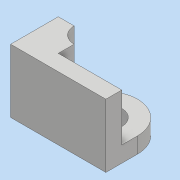
# Autodesk Inventor part: 7
Saved by Autodesk Inventor 2017 (Build 210142000, 142)
## iProperties
Part Number: 7
Material: 一般
Document SubType Name: Modeling
Designer: d8910
Density: 1 g/cm^3
Appearance: 預設
Author: d8910
Autodesk Inventor part; units mm, degrees
ref_plane "YZ Plane" through (0, 0, 0) normal (1, 0, 0) x (0, 1, 0)
ref_plane "XZ Plane" through (0, 0, 0) normal (0, 1, 0) x (-1, 0, 0)
ref_plane "XY Plane" through (0, 0, 0) normal (0, 0, 1) x (1, 0, 0)
sketch "草圖1" plane through (0, 0, 0) normal (0, 1, 0) x (-1, 0, 0)
  line L0 (15, -10) -> (-15, -10)
  line L1 (-15, -10) -> (-15, 10)
  line L2 (-15, 10) -> (15, 10)
  line L3 (15, 10) -> (15, -10)
  point P0 (0, 0)
  point P1 (15, 0)
  point P2 (0, -10)
  dimension "d0" = 30
  dimension "d1" = 20
  constraints: 8 end point, 2 midpoint, 2 parallel, 1 horizontal, 1 horizontal alignment, 1 perpendicular, 1 vertical alignment
  measures "d0" distance of L0.start L0.end
  measures "d1" distance of L2.end L0.start
extrude "擠出1" add sketch "草圖1" along normal blind 5
sketch "草圖2" plane through (15, 0, -10) normal (0, 0, -1) x (-1, 0, 0)
  line L0 (0, 0) -> (30, 0) construction
  line L1 (0, 0) -> (0, 5) construction
  line L2 (30, 5) -> (0, 5) construction
  line L3 (30, 0) -> (30, 5) construction
  line L4 (30, 5) -> (0, 5)
  line L5 (0, 5) -> (0, 10)
  line L6 (30, 10) -> (30, 5)
  arc A0 (20, 10) -> (0, 10) centre (10, 10) ccw
  line L7 (20, 10) -> (30, 10)
  arc A1 (5.3752, 5) -> (14.6248, 5) centre (10, 10) ccw
  circle A2 centre (10, 10) radius 5
  point P0 (15, 0)
  point P1 (0, 7.5)
  dimension "d4" = 20
  dimension "d5" = 5
  dimension "d6" = 5
  dimension "d7" = 10
  dimension "d8" = 10
  constraints: 8 end point, 4 point on circle, 3 centre point, 2 coincident, 2 parallel, 2 point on line, 1 horizontal, 1 midpoint, 1 perpendicular, 1 vertical alignment
  measures "d4" distance from line of L5 L7.start
  measures "d5" distance of L4.end L5.end
  measures "d6" distance of L6.start L2.start
  measures "d7" diameter of A2
  measures "d8" radius of A0
extrude "擠出2" add sketch "草圖2" against normal blind 5 contours L4 L5 A0 L7 L6
sketch "草圖3" plane through (-15, 0, 10) normal (0, 0, 1) x (1, 0, 0)
  line L0 (30, 0) -> (0, 0) construction
  line L1 (30, 0) -> (30, 5) construction
  line L2 (0, 5) -> (30, 5) construction
  line L3 (0, 0) -> (0, 5) construction
  line L4 (0, 0) -> (0, 5) projected
  line L5 (0, 5) -> (10, 5)
  line L6 (10, 5) -> (10, 10)
  line L7 (10, 15) -> (5, 15) construction
  line L8 (0, 15) -> (0, 5)
  arc A0 (5, 15) -> (10, 10) centre (10, 15) ccw
  line L9 (5, 15) -> (0, 15)
  line L10 (10, 10) -> (10, 15) construction
  point P0 (15, 0)
  dimension "d11" = 10
  dimension "d12" = 5
  constraints: 12 end point, 4 parallel, 3 point on circle, 2 perpendicular, 1 centre point, 1 coincident, 1 horizontal
  measures "d11" distance of L7.start L8.start
  measures "d12" radius of A0
extrude "擠出3" add sketch "草圖3" against normal blind 5
